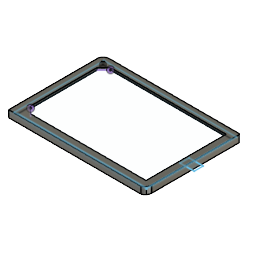
96_wp_deck_i2 (Autodesk Fusion 360 design; units mm, degrees)
part number: 2026-04-28-02-08-20-957
Autodesk Fusion 360 part; units mm, degrees
sketch "Sketch1" plane through (0, 0, 0) normal (0, 0, 1) x (1, 0, 0)
  line L0 (-63.25, 42.05) -> (63.25, 42.05)
  line L1 (63.25, 42.05) -> (63.25, -42.05)
  line L2 (63.25, -42.05) -> (-63.25, -42.05)
  line L3 (-63.25, -42.05) -> (-63.25, 42.05)
  line L4 (0, 42.05) -> (0, -42.05)
  dimension "d5" = 126.5
  dimension "d6" = 84.1
  constraint horizontal L0
  constraint vertical L1
  constraint horizontal L2
  constraint vertical L3
  constraint midpoint L0 L4.start
  constraint midpoint L2 L4.end
  constraint midpoint origin L4
  measures "d5" distance of L0.start L0.end
  measures "d6" distance of L0.start L2.end
extrude "Extrude1" add sketch "Sketch1" along normal blind 3 makes body 1
fillet "Fillet1" radius 1 4 edges at (63.25, 42.05, 1.5) (-63.25, 42.05, 1.5) (-63.25, -42.05, 1.5) (63.25, -42.05, 1.5) on bodies 1
sketch "Sketch2" plane through (0, 0, 3) normal (0, 0, 1) x (-1, 0, 0)
  arc A0 (-62.25, 42.05) -> (-63.25, 41.05) centre (-62.25, 41.05) ccw
  line L0 (-63.25, 41.05) -> (-63.25, -41.05)
  arc A1 (-63.25, -41.05) -> (-62.25, -42.05) centre (-62.25, -41.05) ccw
  line L1 (-62.25, -42.05) -> (62.25, -42.05)
  arc A2 (62.25, -42.05) -> (63.25, -41.05) centre (62.25, -41.05) ccw
  line L2 (63.25, -41.05) -> (63.25, 41.05)
  arc A3 (63.25, 41.05) -> (62.25, 42.05) centre (62.25, 41.05) ccw
  line L3 (62.25, 42.05) -> (-62.25, 42.05)
  line L4 (-10.1311, 42.05) -> (-10.1311, 39.45)
  line L5 (63.25, 39.8442) -> (60.65, 39.8442)
  line L6 (60.65, 39.8442) -> (-61.85, 39.8442)
  line L7 (-61.85, 39.8442) -> (-61.85, -40.2558)
  line L8 (-61.85, -40.2558) -> (60.65, -40.2558)
  line L9 (60.65, -40.2558) -> (60.65, 39.8442)
  dimension "d12" = 2.6
  dimension "d13" = 2.6
  dimension "d16" = 122.5
  dimension "d17" = 80.1
  constraint coincident L3 L4.start
  constraint perpendicular L3 L4
  constraint coincident L2 L5.start
  constraint perpendicular L2 L5
  constraint horizontal L6
  constraint vertical L7
  constraint horizontal L8
  constraint vertical L9
  measures "d12" distance of L4.start L4.end
  measures "d13" distance of L5.start L5.end
extrude "Extrude2" add sketch "Sketch2" along normal blind 12.1 contours L6 L7 L8 L9 bodies 1
chamfer "Chamfer1" distance 6.8 angle 45 2 edges at (-60.65, 40.2558, 9.05) (-60.65, -39.8442, 9.05) on bodies 1
sketch "Sketch3" plane through (0, 0, 3) normal (0, 0, 1) x (-1, 0, 0)
  line L0 (53.85, -40.2558) -> (-61.85, -40.2558)
  line L1 (-61.85, -40.2558) -> (-61.85, 39.8442)
  line L2 (-61.85, 39.8442) -> (53.85, 39.8442)
  line L3 (60.65, 33.0442) -> (60.65, -33.4558)
  arc A0 (-62.25, 42.05) -> (-63.25, 41.05) centre (-62.25, 41.05) ccw
  line L4 (-63.25, 41.05) -> (-63.25, -41.05)
  arc A1 (-63.25, -41.05) -> (-62.25, -42.05) centre (-62.25, -41.05) ccw
  line L5 (-62.25, -42.05) -> (62.25, -42.05)
  arc A2 (62.25, -42.05) -> (63.25, -41.05) centre (62.25, -41.05) ccw
  line L6 (63.25, -41.05) -> (63.25, 41.05)
  arc A3 (63.25, 41.05) -> (62.25, 42.05) centre (62.25, 41.05) ccw
  line L7 (62.25, 42.05) -> (-62.25, 42.05)
  line L8 (62.9571, 41.7571) -> (-63.5429, 41.7571)
  line L9 (-63.5429, 41.7571) -> (-63.5429, -42.7174)
  line L10 (-63.5429, -42.7174) -> (62.9571, -42.3429)
  line L11 (62.9571, -42.3429) -> (62.9571, 41.7571)
  line L12 (60.65, -33.4558) -> (53.85, -40.2558)
  line L13 (53.85, 39.8442) -> (60.65, 33.0442)
  dimension "d22" = 126.5
  dimension "d23" = 84.1
  constraint horizontal L8
  constraint vertical L9
  constraint vertical L11
  constraint midpoint A3 L8.start
  measures "d22" distance of L8.start L8.end
  measures "d23" distance of L8.start L10.end
extrude "Extrude3" add sketch "Sketch3" along normal blind 2 separate body contours A0 L4 A1 L5 A2 L8 L11 makes body 2
move_face "OffsetFaces1" offset 5.5 4 faces at (63.25, -13.6833, 3.6667) (-20.9857, -41.7571, 3.6667) (-62.9571, 13.919, 3.6667) (20.75, 42.05, 3.6667) on bodies 2
sketch "Sketch4" plane through (0, 0, 3) normal (0, 0, -1) x (1, 0, 0)
  arc A0 (67.75, -47.55) -> (68.75, -46.55) centre (67.75, -46.55) ccw
  line L0 (68.75, -46.55) -> (68.75, 41.05)
  arc A1 (68.75, 41.05) -> (64.1792, 47.2571) centre (62.25, 41.05) ccw
  line L1 (64.1792, 47.2571) -> (-68.4571, 47.2571)
  line L2 (-68.4571, 47.2571) -> (-68.4571, -42.9792)
  arc A2 (-68.4571, -42.9792) -> (-62.25, -47.55) centre (-62.25, -41.05) ccw
  line L3 (-62.25, -47.55) -> (67.75, -47.55)
  line L4 (61.85, -40.2558) -> (-53.85, -40.2558)
  line L5 (-60.65, -33.4558) -> (-60.65, 33.0442)
  line L6 (-53.85, 39.8442) -> (61.85, 39.8442)
  line L7 (61.85, 39.8442) -> (61.85, -40.2558)
  line L8 (67.2117, 44.8466) -> (-65.3311, 44.8466)
  line L9 (-65.3311, 44.8466) -> (-65.3311, -45.1406)
  line L10 (-65.3311, -45.1406) -> (67.2117, -45.1406)
  line L11 (67.2117, -45.1406) -> (67.2117, 44.8466)
  line L12 (66.6212, 44.05) -> (-62.25, 44.05)
  line L13 (-62.25, 44.05) -> (-62.25, -41.05)
  line L14 (-62.25, -41.05) -> (66.6212, -41.05)
  line L15 (66.6212, -41.05) -> (66.6212, 44.05)
  line L16 (75.9734, 5.7216) -> (61.8734, 5.7216)
  line L17 (61.8734, 5.7216) -> (61.8734, -3.2784)
  line L18 (61.8734, -3.2784) -> (75.9734, -3.2784)
  line L19 (75.9734, -3.2784) -> (75.9734, 5.7216)
  line L20 (-53.85, -40.2558) -> (-60.65, -33.4558)
  line L21 (-60.65, 33.0442) -> (-53.85, 39.8442)
  dimension "d62" = 14.1
  dimension "d63" = 9
  constraint horizontal L8
  constraint vertical L9
  constraint horizontal L10
  constraint vertical L11
  constraint horizontal L12
  constraint vertical L13
  constraint horizontal L14
  constraint vertical L15
  constraint coincident A2.centre L13.end
  constraint horizontal L16
  constraint vertical L17
  constraint horizontal L18
  constraint vertical L19
  measures "d62" distance of L16.start L16.end
  measures "d63" distance of L16.start L18.end
extrude "Extrude6" add sketch "Sketch4" along normal blind 5 contours A0 L0 A1 L1 L2 A2 L3 L8 L9 L10 L11 L16 L18 | L0 L11 L16 L18 bodies 2
extrude "Extrude7" add sketch "Sketch4" along normal blind 5 contours A0 L0 A1 L1 L2 A2 L3 L8 L9 L10 L11 L16 L18 | L0 L11 L16 L18 bodies 2
extrude "Extrude8" add sketch "Sketch4" along normal blind 1 contours L11 L15 L16 L18 | L8 L9 L10 L11 L12 L13 L14 L15 L16 L18 bodies 2
hidden bodies 1
equation "width = 126.5 mm"
equation "length = 84.1 mm"
equation "base_h = 3.1 mm"
equation "platform_h = 14.1 mm"
equation "d5 = width"
equation "d6 = length"
equation "d7 = top_piece_h"
equation "base_platform_gap = 2.6 mm"
equation "d12 = base_platform_gap"
equation "d13 = base_platform_gap"
equation "platform_width = width - 4 mm"
equation "platform_length = length - 4 mm"
equation "d16 = platform_width"
equation "d17 = platform_length"
equation "platform_shell_depth = 6.8 mm"
equation "d21 = platform_shell_depth"
equation "d22 = width"
equation "d23 = length"
equation "deck_platform_cover_height = 2 mm"
equation "d25 = deck_platform_cover_height"
equation "d27 = deck_base_cover_distance"
equation "deck_base_cover_distance = 5.5 mm"
equation "dmag_6mm = 6.4 mm"
equation "dmag_8mm = 8.4 mm"
equation "dmag_10mm = 10.4 mm"
equation "dmag_thickness = 2.2 mm"
equation "plate_base__depth = 3.3 mm"
equation "top_piece_h = 3 mm"
equation "base_w = 90 mm"
equation "base_l = 131.5 mm"
equation "d47 = base_deck_depth"
equation "weight_incision_l_width = 22 mm"
equation "weight_incision_l_length = 130 mm"
equation "base_deck_depth = 5 mm"
equation "d54 = base_deck_depth"
equation "filling_h = 1 mm"
equation "d57 = filling_h"
equation "clamp_w = 14.1 mm"
equation "clamp_l = 9 mm"
equation "clamp_thickness = 7 mm"
equation "d62 = clamp_w"
equation "d63 = clamp_l"
named bodies: "96wellplate", "deck"
